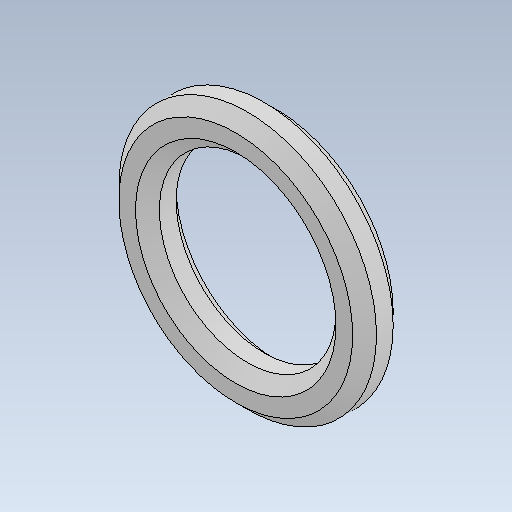
# Autodesk Inventor part: throw-ring
Saved by Autodesk Inventor 2023 (Build 270158030, 158C)
## iProperties
Created: 2024-12-24
Part Number: throw-ring
Material: Generic
Document SubType Name: Modeling
Designer: Imogen Heard
Density: 1 g/cm^3
Appearance: Default
Author: Imogen Heard
Autodesk Inventor part; units mm, degrees
ref_plane "YZ Plane" through (0, 0, 0) normal (1, 0, 0) x (0, 1, 0)
ref_plane "XZ Plane" through (0, 0, 0) normal (0, 1, 0) x (-1, 0, 0)
ref_plane "XY Plane" through (0, 0, 0) normal (0, 0, 1) x (1, 0, 0)
sketch "Sketch1" plane through (0, 0, 0) normal (0, 0, 1) x (1, 0, 0)
  circle A0 centre (17.3511, -55.6305) radius 5.4
  circle A1 centre (17.3511, -55.6305) radius 3.7
  point P0 (0, 0)
  dimension "d0" = 10.8
  dimension "d1" = 1.7
  constraints: 2 centre point
  measures "d0" diameter of A0
  measures "d1" radial gap between concentric circles of A0 A1
extrude "Extrusion1" add sketch "Sketch1" along normal blind 1.7
chamfer "Chamfer1" distance 0.5 angle 45 4 edges at (13.6511, -55.6305, 0) (11.9511, -55.6305, 0) (11.9511, -55.6305, 1.7) (13.6511, -55.6305, 1.7)
body "Solid1"
